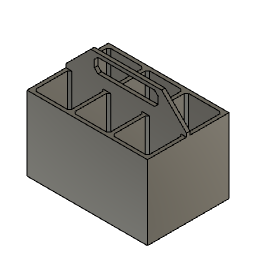
Official Sixpack v3 (Autodesk Fusion 360 design; units mm, degrees)
Autodesk Fusion 360 part; units mm, degrees
sketch "Sketch1" plane through (0, 0, 0) normal (0, 0, 1) x (1, 0, 0)
  line L0 (0, 0) -> (5, 0)
  line L1 (5, 0) -> (5, 5)
  line L2 (5, 5) -> (0, 5)
  line L3 (0, 5) -> (0, 0)
  line L4 (5, 5) -> (5.5, 5) construction
  line L5 (5.5, 5) -> (10.5, 5)
  line L6 (10.5, 5) -> (10.5, 0)
  line L7 (10.5, 0) -> (5.5, 0)
  line L8 (5.5, 0) -> (5.5, 5)
  line L9 (10.5, 5) -> (11, 5) construction
  line L10 (11, 5) -> (16, 5)
  line L11 (16, 5) -> (16, 0)
  line L12 (16, 0) -> (11, 0)
  line L13 (11, 0) -> (11, 5)
  line L14 (0, 5) -> (0, 5.5) construction
  line L15 (0, 5.25) -> (16.5, 5.25) construction
  line L16 (16, 10.5) -> (11, 10.5)
  line L17 (16, 5.5) -> (16, 10.5)
  line L18 (11, 5.5) -> (16, 5.5)
  line L19 (11, 10.5) -> (11, 5.5)
  line L20 (10.5, 5.5) -> (10.5, 10.5)
  line L21 (5.5, 5.5) -> (10.5, 5.5)
  line L22 (10.5, 10.5) -> (5.5, 10.5)
  line L23 (5.5, 10.5) -> (5.5, 5.5)
  line L24 (5, 10.5) -> (5, 5.5)
  line L25 (0, 10.5) -> (5, 10.5)
  line L26 (5, 5.5) -> (0, 5.5)
  line L27 (0, 5.5) -> (0, 10.5)
  line L28 (0, 10.5) -> (-0.5, 10.5) construction
  line L29 (-0.5, 10.5) -> (-0.5, 11) construction
  line L30 (-0.5, 11) -> (16.5, 11)
  line L31 (16.5, 11) -> (16.5, -0.5)
  line L32 (16.5, -0.5) -> (-0.5, -0.5)
  line L33 (-0.5, -0.5) -> (-0.5, 11)
  dimension "d1" = 5
  dimension "d2" = 5
  dimension "d3" = 0.5
  dimension "d4" = 5
  dimension "d5" = 5
  dimension "d6" = 5
  dimension "d7" = 0.5
  dimension "d8" = 0.5
  dimension "d9" = 0.5
  dimension "d10" = 0.5
  dimension "d11" = 17
  dimension "d12" = 11.5
  constraint horizontal L0
  constraint vertical L1
  constraint horizontal L2
  constraint vertical L3
  constraint coincident L0.start L3.end
  constraint perpendicular L1 L4
  constraint horizontal L5
  constraint vertical L6
  constraint horizontal L7
  constraint vertical L8
  constraint perpendicular L6 L9
  constraint horizontal L10
  constraint vertical L11
  constraint horizontal L12
  constraint vertical L13
  constraint perpendicular L2 L14
  constraint midpoint L14 L15.start
  constraint perpendicular L14 L15
  constraint symmetric L0.start L15 L25.start
  constraint symmetric L0.end L15 L24.start
  constraint symmetric L1.end L15 L24.end
  constraint symmetric L2.end L15 L14.end
  constraint symmetric L4.end L15 L21.start
  constraint symmetric L5.end L15 L20.start
  constraint symmetric L6.end L15 L20.end
  constraint symmetric L7.end L15 L22.end
  constraint symmetric L9.end L15 L18.start
  constraint symmetric L10.end L15 L17.start
  constraint symmetric L11.end L15 L16.start
  constraint symmetric L12.end L15 L16.end
  constraint perpendicular L27 L28
  constraint perpendicular L28 L29
  constraint horizontal L30
  constraint vertical L31
  constraint horizontal L32
  constraint vertical L33
  measures "d1" distance of L0.start L0.end
  measures "d2" distance of L0.start L2.end
  measures "d3" distance of L1.end L4.end
  measures "d4" distance of L4.end L5.end
  measures "d5" distance of L9.end L10.end
  measures "d6" distance of L10.end L11.end
  measures "d7" distance of L5.end L9.end
  measures "d8" distance of L2.end L14.end
  measures "d9" distance of L25.start L28.end
  measures "d10" distance of L28.end L29.end
  measures "d11" distance of L29.end L30.end
  measures "d12" distance of L29.end L32.end
extrude "Extrude1" add sketch "Sketch1" along normal blind 10 makes body 1
chamfer "Chamfer1" distance 0.3 angle 45 23 edges at (0, 5, 5) (0, 10.5, 5) (5.5, 5, 5) (5.5, 10.5, 5) (11, 5, 5) (11, 10.5, 5) (0, 5.5, 5) (0, 0, 5) (5, 0, 5) (5, 5, 5) (11, 0, 5) (16, 5, 5) (16, 10.5, 5) (16, 0, 5) (10.5, 5.5, 5) (16, 5.5, 5) (10.5, 0, 5) (5, 5.5, 5) (5.5, 5.5, 5) (11, 5.5, 5) (10.5, 5, 5) (10.5, 10.5, 5) (5, 10.5, 5) on bodies 1
sketch "Sketch2" plane through (0, 0, 0) normal (0, 0, -1) x (1, 0, 0)
  line L0 (4.7, -5.5) -> (5, -5.8)
  line L1 (5, -5.8) -> (5, -10.2)
  line L2 (5, -10.2) -> (4.7, -10.5)
  line L3 (4.7, -10.5) -> (0.3, -10.5)
  line L4 (0.3, -10.5) -> (0, -10.2)
  line L5 (0, -10.2) -> (0, -5.8)
  line L6 (0, -5.8) -> (0.3, -5.5)
  line L7 (0.3, -5.5) -> (4.7, -5.5)
  line L8 (0, -0.3) -> (0.3, 0)
  line L9 (0.3, 0) -> (4.7, 0)
  line L10 (4.7, 0) -> (5, -0.3)
  line L11 (5, -0.3) -> (5, -4.7)
  line L12 (5, -4.7) -> (4.7, -5)
  line L13 (4.7, -5) -> (0.3, -5)
  line L14 (0.3, -5) -> (0, -4.7)
  line L15 (0, -4.7) -> (0, -0.3)
  line L16 (10.2, 0) -> (10.5, -0.3)
  line L17 (10.5, -0.3) -> (10.5, -4.7)
  line L18 (10.5, -4.7) -> (10.2, -5)
  line L19 (10.2, -5) -> (5.8, -5)
  line L20 (5.8, -5) -> (5.5, -4.7)
  line L21 (5.5, -4.7) -> (5.5, 0)
  line L22 (5.5, 0) -> (10.2, 0)
  line L23 (5.5, -5.8) -> (5.8, -5.5)
  line L24 (5.8, -5.5) -> (10.2, -5.5)
  line L25 (10.2, -5.5) -> (10.5, -5.8)
  line L26 (10.5, -5.8) -> (10.5, -10.2)
  line L27 (10.5, -10.2) -> (10.2, -10.5)
  line L28 (10.2, -10.5) -> (5.8, -10.5)
  line L29 (5.8, -10.5) -> (5.5, -10.2)
  line L30 (5.5, -10.2) -> (5.5, -5.8)
  line L31 (11, -5.8) -> (11.3, -5.5)
  line L32 (11.3, -5.5) -> (15.7, -5.5)
  line L33 (15.7, -5.5) -> (16, -5.8)
  line L34 (16, -5.8) -> (16, -10.2)
  line L35 (16, -10.2) -> (15.7, -10.5)
  line L36 (15.7, -10.5) -> (11.3, -10.5)
  line L37 (11.3, -10.5) -> (11, -10.2)
  line L38 (11, -10.2) -> (11, -5.8)
  line L39 (15.7, 0) -> (16, -0.3)
  line L40 (16, -0.3) -> (16, -4.7)
  line L41 (16, -4.7) -> (15.7, -5)
  line L42 (15.7, -5) -> (11.3, -5)
  line L43 (11.3, -5) -> (11, -4.7)
  line L44 (11, -4.7) -> (11, -0.3)
  line L45 (11, -0.3) -> (11.3, 0)
  line L46 (11.3, 0) -> (15.7, 0)
  line L47 (16.5, 0.5) -> (-0.5, 0.5)
  line L48 (-0.5, 0.5) -> (-0.5, -11)
  line L49 (-0.5, -11) -> (16.5, -11)
  line L50 (16.5, -11) -> (16.5, 0.5)
  line L51 (16.5, -11) -> (-0.5, -11)
  line L52 (-0.5, -11) -> (-0.5, 0.5)
  line L53 (-0.5, 0.5) -> (16.5, 0.5)
  line L54 (16.5, 0.5) -> (16.5, -11)
  constraint horizontal L51
  constraint vertical L52
  constraint horizontal L53
  constraint vertical L54
  constraint coincident L47.end L48.start
  constraint coincident L49.end L50.start
extrude "Extrude2" add sketch "Sketch2" along normal blind 0.5 contours L0 L1 L2 L3 L4 L5 L6 L7 | L8 L9 L10 L11 L12 L13 L14 L15 | L16 L17 L18 L19 L20 L21 L22 | L23 L24 L25 L26 L27 L28 L29 L30 | L31 L32 L33 L34 L35 L36 L37 L38 | L39 L40 L41 L42 L43 L44 L45 L46 | L47 L48 L49 L50 L51 L52 L53 L54 bodies 1
sketch "Sketch3" plane through (0, 0, 10) normal (0, 0, 1) x (-1, 0, 0)
  line L0 (-4.7, -5.5) -> (-0.3, -5.5)
  line L1 (-0.3, -5.5) -> (0, -5.8)
  line L2 (0, -5.8) -> (0, -10.2)
  line L3 (0, -10.2) -> (-0.3, -10.5)
  line L4 (-0.3, -10.5) -> (-4.7, -10.5)
  line L5 (-4.7, -10.5) -> (-5, -10.2)
  line L6 (-5, -10.2) -> (-5, -5.8)
  line L7 (-5, -5.8) -> (-4.7, -5.5)
  line L8 (0, -0.3) -> (0, -4.7)
  line L9 (0, -4.7) -> (-0.3, -5)
  line L10 (-0.3, -5) -> (-4.7, -5)
  line L11 (-4.7, -5) -> (-5, -4.7)
  line L12 (-5, -4.7) -> (-5, -0.3)
  line L13 (-5, -0.3) -> (-4.7, 0)
  line L14 (-4.7, 0) -> (-0.3, 0)
  line L15 (-0.3, 0) -> (0, -0.3)
  line L16 (-10.2, 0) -> (-5.5, 0)
  line L17 (-5.5, 0) -> (-5.5, -4.7)
  line L18 (-5.5, -4.7) -> (-5.8, -5)
  line L19 (-5.8, -5) -> (-10.2, -5)
  line L20 (-10.2, -5) -> (-10.5, -4.7)
  line L21 (-10.5, -4.7) -> (-10.5, -0.3)
  line L22 (-10.5, -0.3) -> (-10.2, 0)
  line L23 (-5.5, -5.8) -> (-5.5, -10.2)
  line L24 (-5.5, -10.2) -> (-5.8, -10.5)
  line L25 (-5.8, -10.5) -> (-10.2, -10.5)
  line L26 (-10.2, -10.5) -> (-10.5, -10.2)
  line L27 (-10.5, -10.2) -> (-10.5, -5.8)
  line L28 (-10.5, -5.8) -> (-10.2, -5.5)
  line L29 (-10.2, -5.5) -> (-5.8, -5.5)
  line L30 (-5.8, -5.5) -> (-5.5, -5.8)
  line L31 (-11, -5.8) -> (-11, -10.2)
  line L32 (-11, -10.2) -> (-11.3, -10.5)
  line L33 (-11.3, -10.5) -> (-15.7, -10.5)
  line L34 (-15.7, -10.5) -> (-16, -10.2)
  line L35 (-16, -10.2) -> (-16, -5.8)
  line L36 (-16, -5.8) -> (-15.7, -5.5)
  line L37 (-15.7, -5.5) -> (-11.3, -5.5)
  line L38 (-11.3, -5.5) -> (-11, -5.8)
  line L39 (-15.7, 0) -> (-11.3, 0)
  line L40 (-11.3, 0) -> (-11, -0.3)
  line L41 (-11, -0.3) -> (-11, -4.7)
  line L42 (-11, -4.7) -> (-11.3, -5)
  line L43 (-11.3, -5) -> (-15.7, -5)
  line L44 (-15.7, -5) -> (-16, -4.7)
  line L45 (-16, -4.7) -> (-16, -0.3)
  line L46 (-16, -0.3) -> (-15.7, 0)
  line L47 (0.5, 0.5) -> (-16.5, 0.5)
  line L48 (-16.5, 0.5) -> (-16.5, -11)
  line L49 (-16.5, -11) -> (0.5, -11)
  line L50 (0.5, -11) -> (0.5, 0.5)
  line L51 (-16.5, -5) -> (0.5, -5)
  line L52 (0.5, -5) -> (0.5, -5.5)
  line L53 (0.5, -5.5) -> (-16.5, -5.5)
  line L54 (-16.5, -5.5) -> (-16.5, -5)
  dimension "d18" = 17
  dimension "d19" = 0.5
  constraint horizontal L51
  constraint vertical L52
  constraint horizontal L53
  constraint vertical L54
  constraint coincident L48 L51.start
  measures "d18" distance of L51.start L51.end
  measures "d19" distance of L51.start L53.end
extrude "Extrude3" add sketch "Sketch3" along normal blind 4 contours L0 L10 L19 L29 L37 L43 L48 L50 L51 L52 L53 L54 bodies 1
chamfer "Chamfer2" distance 0.3 angle 45 1 edges at (5.5, 0, 5) on bodies 1
chamfer "Chamfer3" distance 3.5 angle 45 2 edges at (16.5, 5.25, 14) (-0.5, 5.25, 14) on bodies 1
sketch "Sketch4" plane through (0, 5.5, 0) normal (0, 1, 0) x (-1, 0, 0)
  line L0 (0.5, 10.5) -> (-3, 14)
  line L1 (-3, 14) -> (-13, 14)
  line L2 (-13, 14) -> (-16.5, 10.5)
  line L3 (-16.5, 10.5) -> (-16.5, 10)
  line L4 (-16.5, 10) -> (-15.7, 10)
  line L5 (-15.7, 10) -> (-15.7, 0)
  line L6 (-15.7, 0) -> (-11.3, 0)
  line L7 (-11.3, 0) -> (-11.3, 10)
  line L8 (-11.3, 10) -> (-10.2, 10)
  line L9 (-10.2, 10) -> (-10.2, 0)
  line L10 (-10.2, 0) -> (-5.8, 0)
  line L11 (-5.8, 0) -> (-5.8, 10)
  line L12 (-5.8, 10) -> (-4.7, 10)
  line L13 (-4.7, 10) -> (-4.7, 0)
  line L14 (-4.7, 0) -> (-0.3, 0)
  line L15 (-0.3, 0) -> (-0.3, 10)
  line L16 (-0.3, 10) -> (0.5, 10)
  line L17 (0.5, 10) -> (0.5, 10.5)
  line L18 (-12.5, 13.5) -> (-3.5, 13.5)
  line L19 (-12.5, 13.5) -> (-3.5, 13.5)
  line L20 (-3.5, 13.5) -> (-3.5, 11.5)
  line L21 (-3.5, 11.5) -> (-12.5, 11.5)
  line L22 (-12.5, 11.5) -> (-12.5, 13.5)
  line L23 (-12.5, 12) -> (-12, 11.5)
  line L24 (-12.5, 13) -> (-12, 13.5)
  line L25 (-4, 13.5) -> (-3.5, 13)
  line L26 (-3.5, 12) -> (-4, 11.5)
  constraint horizontal L18
  constraint horizontal L19
  constraint vertical L20
  constraint horizontal L21
  constraint vertical L22
  constraint coincident L22 L23.start
  constraint coincident L21 L23.end
  constraint coincident L22 L24.start
  constraint coincident L18 L24.end
  constraint perpendicular L23 L24
  constraint coincident L18 L25.start
  constraint coincident L20 L25.end
  constraint perpendicular L24 L25
  constraint coincident L20 L26.start
  constraint coincident L21 L26.end
  constraint perpendicular L25 L26
extrude "Extrude4" cut sketch "Sketch4" against normal up to surface (0.5 mm away) contours L18 L19 L20 L21 L22 L23 L24 L25 L26 bodies 1
scale "Scale1" factor 2.352 about (16, 10.2, 10) bodies 1
copy_body "Body->Comp1" bodies 1 removing the originals makes body 2 in component "Component"
component "Component" placed x (1, 0, 0) y (0, 1, 0) z (0, 0, 1) at (0, 0, 0)
